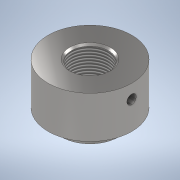
# Autodesk Inventor part: Гайка шток-поршень
Saved by Autodesk Inventor 2021 (Build 250183000, 183)
## iProperties
Created: 2020-11-21
Part Number: Гайка шток-поршень
Material: Сталь, углеродистая
Document SubType Name: Modeling
Designer: Тимоха
Mass: 1999.67 g
Surface Area: 319.942 cm^2
Volume: 254.735 cm^3
Density: 7.85 g/cm^3
Appearance: С умеренной полировкой
Author: Тимоха
Autodesk Inventor part; units mm, degrees
ref_plane "YZ Plane" through (0, 0, 0) normal (1, 0, 0) x (0, 1, 0)
ref_plane "XZ Plane" through (0, 0, 0) normal (0, 1, 0) x (-1, 0, 0)
ref_plane "XY Plane" through (0, 0, 0) normal (0, 0, 1) x (1, 0, 0)
sketch "Эскиз1" plane through (0, 0, 0) normal (0, 0, 1) x (1, 0, 0)
  line L0 (0, 0) -> (45, 0)
  line L1 (45, 0) -> (45, -45)
  line L2 (45, -45) -> (35, -45)
  line L3 (20, -65) -> (20, 0)
  line L4 (35, -45) -> (27.6938, -65.0737)
  line L5 (20, -57.4838) -> (30.4563, -57.4838)
  line L6 (0, 0) -> (0, -13.3093)
  dimension "d0" = 45
  dimension "d1" = 45
  dimension "d2" = 10
  dimension "d5" = 20
  dimension "d6" = 110
  constraints: 14 end point, 2 horizontal, 2 perpendicular, 2 point on line, 2 vertical
  measures "d0" distance of L0.start L0.end
  measures "d1" distance of L0.end L1.end
  measures "d2" distance of L1.end L2.end
  measures "d5" distance from line of L0.start L3
  measures "d6" angle of L0 L4
revolve "Вращение1" add sketch "Эскиз1" angle 360 about axis through (0, 0, 0) along (0, -1, 0)
thread "Резьба1" size "M40x3" class "6H" standard "ANSI Metric M Profile" full length
chamfer "Фаска1" distance 2 angle 45 2 edges at (-20, 0, 0) (-20, -57.4838, 0)
sketch "Эскиз2" plane through (0, 0, 0) normal (0, 0, 1) x (1, 0, 0)
  line L0 (45, 0) -> (45, -45) projected
  line L1 (45, 0) -> (45, -15)
  line L2 (45, -15) -> (34.4215, -15)
  line L3 (45, -15) -> (45, -10)
  line L4 (45, -10) -> (35, -10)
  line L5 (35, -10) -> (31.8757, -15)
  line L6 (34.4215, -15) -> (31.8757, -15)
  point P0 (0, 0)
  dimension "d13" = 15
  dimension "d14" = 5
  dimension "d15" = 10
  dimension "d17" = 58
  constraints: 12 end point, 3 point on line, 2 perpendicular, 1 horizontal
  measures "d13" distance of L1.start L1.end
  measures "d14" distance of L1.end L3.end
  measures "d15" distance of L3.end L4.end
  measures "d17" angle of L2 L5
revolve "Вращение2" cut sketch "Эскиз2" angle 360 about axis through (45, -15, 0) along (-1, 0, 0)
